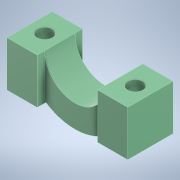
# Autodesk Inventor part: 连接下环
Saved by Autodesk Inventor 2022 (Build 260153000, 153)
## iProperties
Created: 2023-02-21
Part Number: 连接下环
Material: 常规
Document SubType Name: Modeling
Designer: 李承轩
Density: 1 g/cm^3
Appearance: 平滑 - 深海绿色
Author: 李承轩
Autodesk Inventor part; units mm, degrees
ref_plane "YZ Plane" through (0, 0, 0) normal (1, 0, 0) x (0, 1, 0)
ref_plane "XZ Plane" through (0, 0, 0) normal (0, 1, 0) x (-1, 0, 0)
ref_plane "XY Plane" through (0, 0, 0) normal (0, 0, 1) x (1, 0, 0)
sketch "草图1" plane through (0, 0, 0) normal (0, 0, 1) x (1, 0, 0)
  circle A0 centre (0, 0) radius 20 projected
  circle A1 centre (0, 0) radius 35
  line L0 (-35, 0) -> (35, 0)
  point P0 (-20, 0)
  point P1 (20, 0)
  dimension "d0" = 70
  dimension "d1" = 70
  constraints: 2 end point, 2 point on circle, 1 centre point, 1 coincident, 1 horizontal
  measures "d0" diameter of A1
  measures "d1" distance of L0.start L0.end
extrude "拉伸1" add sketch "草图1" along normal mid plane 20 contours L0 A1 A0 picked at (-29.7075, -2.5961)
sketch "草图2" plane through (0, 0, 0) normal (0, 0, 1) x (1, 0, 0)
  line L0 (-20, 0) -> (-40, 0)
  line L1 (-40, 0) -> (-40, -30)
  line L2 (-40, -30) -> (-20, -30)
  line L3 (-20, -30) -> (-20, 0)
  line L4 (20, 0) -> (35, 0) projected
  line L5 (20, 0) -> (40, 0)
  line L6 (40, 0) -> (40, -30)
  line L7 (40, -30) -> (20, -30)
  line L8 (20, -30) -> (20, 0)
  point P0 (0, 0)
  dimension "d4" = 20
  dimension "d5" = 30
  dimension "d6" = 20
  dimension "d7" = 30
  constraints: 16 end point, 4 parallel, 2 horizontal, 2 perpendicular
  measures "d4" distance of L2.end L1.end
  measures "d5" distance of L1.end L0.end
  measures "d6" distance of L6.end L7.end
  measures "d7" distance of L5.end L6.end
extrude "拉伸2" add sketch "草图2" along normal mid plane 30
sketch "草图3" plane through (-40, 0, -15) normal (0, 1, 0) x (1, 0, 0)
  line L0 (20, -5) -> (20, -25) construction
  line L1 (20, 0) -> (20, -5) construction
  line L2 (0, 0) -> (20, 0) construction
  line L3 (0, -30) -> (0, 0) construction
  line L4 (20, -30) -> (0, -30) construction
  line L5 (20, -25) -> (20, -30) construction
  point P0 (40, -15)
  point P1 (10, -15)
  point P2 (20, -15)
  point P3 (10, 0)
  constraints: 2 midpoint, 1 horizontal alignment, 1 vertical alignment
hole "孔1" at (-30, 0, 0) direction (0, -1, 0) diameter 10 end through all
mirror "镜像1" about plane through (0, 0, 0) normal (1, 0, 0) of "孔1"
